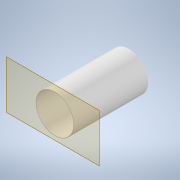
# Autodesk Inventor part: motor_vtulka
Saved by Autodesk Inventor 2022 (Build 260153000, 153)
## iProperties
Created: 2024-12-11
Part Number: motor_vtulka
Material: Типовые
Document SubType Name: Modeling
Designer: Andrey
Density: 1 g/cm^3
Appearance: По умолчанию
Author: Andrey
Autodesk Inventor part; units mm, degrees
ref_plane "YZ Plane" through (0, 0, 0) normal (1, 0, 0) x (0, 1, 0)
ref_plane "XZ Plane" through (0, 0, 0) normal (0, 1, 0) x (-1, 0, 0)
ref_plane "РабПлоскость1" through (0, 0, 0) normal (0, 0, 1) x (1, 0, 0)
ref_plane "РабПлоскость2" through (-62.145235, -0.948385, -51) normal (0, 0, -1) x (0.0152604, 0.9998836, 0)
sketch "Эскиз1" plane through (0, 0, 0) normal (0, 0, 1) x (1, 0, 0)
  circle A0 centre (-49.146748, -0.75) radius 13
  arc A1 (-26.791374, 12.735328) -> (-27.346776, 13.802246) centre (-28.76099, 12.388032) ccw
  line L0 (-27.346776, 13.802246) -> (-28.294531, 14.75)
  line L1 (-28.294531, 14.75) -> (-49.146748, 14.75)
  arc A2 (-49.146748, 14.75) -> (-61.552305, 8.542586) centre (-49.146748, -0.75) ccw
  line L2 (-61.552305, 8.542586) -> (-79, -14.75)
  line L3 (-79, -14.75) -> (-21.944969, -14.75)
  line L4 (-21.944969, -14.75) -> (-26.302484, 9.962691)
  line L5 (-26.302484, 9.962691) -> (-32.5, 9.962691)
  line L6 (-32.5, 9.962691) -> (-32.5, 12.162691)
  line L7 (-32.5, 12.162691) -> (-26.690403, 12.162691)
  line L8 (-26.690403, 12.162691) -> (-26.791374, 12.735328)
  circle A3 centre (-36.5, 10.75) radius 2.1
  circle A4 centre (-29.57484, -8.75) radius 2.1
  circle A5 centre (-67.146748, -8.75) radius 2.1
  circle A6 centre (-72.089282, -11.292059) radius 3.05
  circle A7 centre (-49.146748, -0.75) radius 12.9
  circle A8 centre (-49.146748, -0.75) radius 12.6
  point P0 (0, 0)
  dimension "d0" = 0.1
  dimension "d1" = 0.3
  constraints: 2 centre point
  measures "d0" radial gap between concentric circles of A0 A7
  measures "d1" radial gap between concentric circles of A7 A8
sketch "Эскиз1 outline for Выдавливание1" plane through (0, 0, 0) normal (0, 0, 1) x (1, 0, 0)
  circle A0 centre (-49.146748, -0.75) radius 12.9
  circle A1 centre (-49.146748, -0.75) radius 12.6
extrude "Выдавливание1" add sketch "Эскиз1 outline for Выдавливание1" against normal up to surface (51 mm away)
